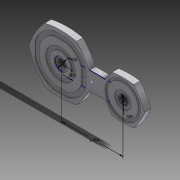
# Autodesk Inventor part: Frame
Saved by Autodesk Inventor 2018 (Build 220112000, 112)
## iProperties
Created: 2018-01-20
Part Number: Frame
Material: ABS Plastic
Document SubType Name: Modeling
Designer: Rus
Density: 1.06 g/cm^3
Appearance: Smooth - White
Author: Rus
Autodesk Inventor part; units mm, degrees
ref_plane "YZ Plane" through (0, 0, 0) normal (1, 0, 0) x (0, 1, 0)
ref_plane "XZ Plane" through (0, 0, 0) normal (0, 1, 0) x (-1, 0, 0)
ref_plane "XY Plane" through (0, 0, 0) normal (0, 0, 1) x (1, 0, 0)
sketch "Sketch1" plane through (0, 0, 0) normal (0, 0, 1) x (1, 0, 0)
  circle A0 centre (-43.9941, 0) radius 9.525
  circle A1 centre (43.9941, 0) radius 6.35
  line L0 (43.9941, 0) -> (-43.9941, 0) construction
  line L1 (43.9941, 12.7) -> (-43.9941, 12.7)
  line L2 (-43.9941, -12.7) -> (43.9941, -12.7)
  arc A2 (43.9941, -12.7) -> (43.9941, 12.7) centre (43.9941, 0) ccw
  arc A3 (-43.9941, 12.7) -> (-43.9941, -12.7) centre (-43.9941, 0) ccw
  point P0 (0, 0)
  point P1 (0, 0)
  dimension "d10" = 12.7
  dimension "d11" = 19.05
  dimension "d12" = 87.9881
  dimension "d13" = 12.7
  constraints: 8 end point, 4 centre point, 4 point on circle, 4 tangent, 1 coincident, 1 horizontal, 1 midpoint, 1 parallel
  measures "d10" diameter of A1
  measures "d11" diameter of A0
  measures "d12" distance of L0.start L0.end
  measures "d13" distance of L2.start L0.end
sketch "Sketch3" plane through (0, 0, 0) normal (0, 0, 1) x (1, 0, 0)
  line L0 (-44.9008, 0) -> (44.9008, 0) construction
  line L1 (-44.9008, -12.7) -> (44.9008, -12.7)
  line L2 (44.9008, 12.7) -> (-44.9008, 12.7)
  arc A0 (-44.9008, 12.7) -> (-44.9008, -12.7) centre (-44.9008, 0) ccw
  arc A1 (44.9008, -12.7) -> (44.9008, 12.7) centre (44.9008, 0) ccw
  circle A2 centre (-44.9008, 0) radius 6.35
  point P0 (0, 0)
  dimension "d23" = 44.9008
  dimension "d24" = 25.4
  dimension "d25" = 12.7
  constraints: 8 end point, 4 point on circle, 4 tangent, 3 centre point, 1 coincident, 1 horizontal, 1 midpoint, 1 parallel
  measures "d23" distance of point (0, 0) L0.end
  measures "d24" distance between parallel lines of L1 L2
  measures "d25" diameter of A2
extrude "Extrusion4" add sketch "Sketch3" against normal blind 8.4667
sketch "Sketch4" plane through (0, 0, -8.4667) normal (0, 0, -1) x (-1, 0, 0)
  circle A0 centre (-44.9008, 0) radius 6.35
  arc A1 (-44.9008, 12.7) -> (-44.9008, -12.7) centre (-44.9008, 0) ccw projected
  point P0 (0, 0)
  dimension "d28" = 12.7
  constraints: 1 centre point, 1 coincident
  measures "d28" diameter of A0
extrude "Extrusion5" cut sketch "Sketch4" against normal through all
sketch "Sketch5" plane through (0, 0, -8.4667) normal (0, 0, -1) x (-1, 0, 0)
  circle A0 centre (44.9008, 0) radius 6.35 projected
  line L0 (67.7609, 39.5947) -> (90.6209, 0)
  line L1 (90.6209, 0) -> (67.7608, -39.5947)
  line L2 (67.7608, -39.5947) -> (22.0408, -39.5947)
  line L3 (22.0408, -39.5947) -> (-0.8192, 0)
  line L4 (-0.8192, 0) -> (22.0409, 39.5947)
  line L5 (22.0409, 39.5947) -> (67.7609, 39.5947)
  line L6 (-44.9008, 12.7) -> (44.9008, 12.7) projected
  point P0 (0, 0)
  dimension "d31" = 45.72
  constraints: 12 end point, 2 coincident, 1 parallel, 13 other
  measures "d31" distance of L4.end L0.start
extrude "Extrusion6" add sketch "Sketch5" against normal up to surface (8.4667 mm away)
sketch "Sketch6" plane through (0, 0, 0) normal (0, 0, 1) x (1, 0, 0)
  line L0 (-52.1227, 63.088) -> (-51.6134, 26.2115) projected
  arc A0 (-51.6134, 26.2115) -> (-38.9146, 26.3869) centre (-45.264, 26.2992) ccw projected
  line L1 (-38.9146, 26.3869) -> (-39.4239, 63.2634) projected
  arc A1 (-26.5904, 60.8028) -> (-39.4239, 63.2634) centre (-44.9009, 0) ccw projected
  arc A2 (-26.5904, 60.8028) -> (15.3735, 19.9814) centre (17.7163, 64.3696) ccw projected
  arc A3 (18.1873, 7.2206) -> (15.3735, 19.9814) centre (-44.9009, 0) ccw projected
  line L2 (18.1873, 7.2206) -> (-18.6893, 6.7126) projected
  arc A4 (-18.6893, 6.7126) -> (-18.514, -5.9862) centre (-18.6017, 0.3632) ccw projected
  line L3 (-18.514, -5.9862) -> (18.3625, -5.4769) projected
  arc A5 (15.9019, -18.3105) -> (18.3625, -5.4769) centre (-44.9009, 0) ccw projected
  arc A6 (15.9019, -18.3105) -> (-24.9195, -60.2743) centre (19.4687, -62.6171) ccw projected
  arc A7 (-37.679, -63.088) -> (-24.9195, -60.2743) centre (-44.9009, 0) ccw projected
  line L4 (-37.679, -63.088) -> (-38.1883, -26.2115) projected
  arc A8 (-38.1883, -26.2115) -> (-50.8871, -26.3869) centre (-44.5377, -26.2992) ccw projected
  line L5 (-50.8871, -26.3869) -> (-50.3778, -63.2634) projected
  arc A9 (-63.2113, -60.8028) -> (-50.3778, -63.2634) centre (-44.9009, 0) ccw projected
  arc A10 (-63.2113, -60.8028) -> (-105.1752, -19.9814) centre (-107.518, -64.3696) ccw projected
  arc A11 (-107.9888, -7.2218) -> (-105.1752, -19.9814) centre (-44.9009, 0) ccw projected
  line L6 (-107.9888, -7.2218) -> (-71.1124, -6.7126) construction
  arc A12 (-71.1124, -6.7126) -> (-71.2877, 5.9862) centre (-71.2, -0.3632) ccw projected
  line L7 (-71.2877, 5.9862) -> (-108.1642, 5.4769) projected
  arc A13 (-105.7036, 18.3105) -> (-108.1642, 5.4769) centre (-44.9009, 0) ccw projected
  arc A14 (-105.7036, 18.3105) -> (-64.8822, 60.2743) centre (-109.2704, 62.6171) ccw projected
  arc A15 (-52.1227, 63.088) -> (-64.8822, 60.2743) centre (-44.9009, 0) ccw projected
  arc A16 (-55.6968, 34.5475) -> (-79.7331, 9.8384) centre (-44.9009, 0) ccw projected
  arc A17 (-79.7331, 9.8384) -> (-78.5109, 9.4932) centre (-79.122, 9.6658) ccw projected
  arc A18 (-55.318, 33.3353) -> (-78.5109, 9.4932) centre (-44.9009, 0) ccw projected
  arc A19 (-55.318, 33.3353) -> (-55.6968, 34.5475) centre (-55.5074, 33.9414) ccw projected
  arc A20 (-79.4483, -10.7959) -> (-54.7393, -34.8322) centre (-44.9009, 0) ccw projected
  arc A21 (-54.7393, -34.8322) -> (-54.3941, -33.61) centre (-54.5667, -34.2211) ccw projected
  arc A22 (-78.2361, -10.4171) -> (-54.3941, -33.61) centre (-44.9009, 0) ccw projected
  arc A23 (-78.2361, -10.4171) -> (-79.4483, -10.7959) centre (-78.8422, -10.6065) ccw projected
  arc A24 (-34.1049, -34.5475) -> (-10.0686, -9.8384) centre (-44.9009, 0) ccw projected
  arc A25 (-10.0686, -9.8384) -> (-11.2908, -9.4932) centre (-10.6797, -9.6658) ccw projected
  arc A26 (-34.4837, -33.3353) -> (-11.2908, -9.4932) centre (-44.9009, 0) ccw projected
  arc A27 (-34.4837, -33.3353) -> (-34.1049, -34.5475) centre (-34.2943, -33.9414) ccw projected
  arc A28 (-10.3534, 10.7959) -> (-35.0624, 34.8322) centre (-44.9009, 0) ccw projected
  arc A29 (-35.0624, 34.8322) -> (-35.4076, 33.61) centre (-35.235, 34.2211) ccw projected
  arc A30 (-11.5656, 10.4171) -> (-35.4076, 33.61) centre (-44.9009, 0) ccw projected
  arc A31 (-11.5656, 10.4171) -> (-10.3534, 10.7959) centre (-10.9595, 10.6065) ccw projected
  circle A32 centre (-44.9009, 0) radius 19.05 projected
  line L8 (-22.0408, -39.5947) -> (-67.7608, -39.5947) projected
  line L9 (-67.7609, -39.5947) -> (-90.6209, 0)
  line L10 (-90.6209, 0) -> (-67.7609, 39.5947)
  line L11 (-67.7609, 39.5947) -> (-22.0409, 39.5947)
  line L12 (-22.0409, 39.5947) -> (0.8191, 0)
  line L13 (0.8191, 0) -> (-22.0409, -39.5947)
  line L14 (-22.0409, -39.5947) -> (-67.7609, -39.5947)
  circle A33 centre (-44.9009, 0) radius 15.875
  circle A34 centre (-44.9009, 0) radius 17.78 projected
  circle A35 centre (-44.9009, 0) radius 9.525
  arc A36 (-54.7619, 36.8018) -> (-81.7026, 9.861) centre (-44.9009, 0) ccw
  line L15 (-44.9009, 0) -> (-71.8416, 26.9408) construction
  line L16 (-44.9009, 0) -> (-17.9601, 26.9408) construction
  arc A37 (-8.0991, 9.861) -> (-35.0398, 36.8018) centre (-44.9009, 0) ccw
  line L17 (-44.9009, 0) -> (-35.0398, 36.8018) construction
  line L18 (-44.9009, 0) -> (-6.8009, 0) construction
  line L19 (-54.7619, 36.8018) -> (-35.0398, 36.8018)
  line L20 (-67.7608, -39.5947) -> (-90.6209, 0) construction
  line L21 (-44.9009, 36.8018) -> (-90.6209, 0) construction
  line L22 (-81.7026, 9.861) -> (-81.5664, 0)
  line L23 (-44.9009, 0) -> (-81.5664, 0) construction
  line L24 (-8.0991, 9.861) -> (-8.0991, 0)
  arc A38 (-81.7026, -9.861) -> (-54.7619, -36.8018) centre (-44.9009, 0) ccw
  arc A39 (-35.0398, -36.8018) -> (-8.0991, -9.861) centre (-44.9009, 0) ccw
  line L25 (-54.7619, -36.8018) -> (-35.0398, -36.8018)
  line L26 (-81.7026, -9.861) -> (-81.5664, 0)
  line L27 (-8.0991, -9.861) -> (-8.0991, 0)
  circle A40 centre (-44.9009, 0) radius 21.1667
  arc A41 (-75.9187, -6.779) -> (-75.1884, -9.525) centre (-44.9009, 0) ccw construction
  line L28 (-75.1884, -9.525) -> (-75.1884, 9.525)
  line L29 (-54.4259, 30.2876) -> (-35.3758, 30.2876)
  line L30 (-14.6133, 9.525) -> (-14.6133, -9.525)
  line L31 (-35.3759, -30.2876) -> (-54.4259, -30.2876)
  arc A42 (-81.7026, 9.861) -> (-81.7026, -9.861) centre (-44.9009, 0) ccw construction
  line L32 (-76.6509, 0) -> (-75.1884, 0) construction
  arc A43 (-76.6509, 0) -> (-75.9187, -6.779) centre (-44.9009, 0) ccw construction
  arc A44 (-75.1884, -9.525) -> (-75.1884, 9.525) centre (-44.9009, 0) ccw
  arc A45 (-76.0941, 5.9198) -> (-76.6509, 0) centre (-44.9009, 0) ccw construction
  arc A46 (-75.1884, 9.525) -> (-76.0941, 5.9198) centre (-44.9009, 0) ccw
  point P0 (0, 0)
  point P1 (-44.9008, -39.5947)
  dimension "d43" = 63.5
  dimension "d34" = 31.75
  dimension "d35" = 19.05
  dimension "d36" = 60
  dimension "d37" = 38.1
  dimension "d38" = 38.1
  dimension "d40" = 60
  dimension "d41" = 90
  dimension "d42" = 42.3333
  dimension "d44" = 19.05
  dimension "d45" = 19.05
  constraints: 46 end point, 30 point on circle, 11 centre point, 9 coincident, 5 point on line, 4 horizontal, 4 midpoint, 4 symmetric about line, 3 equal length, 3 perpendicular, 2 parallel, 37 other
  measures "d34" diameter of A33
  measures "d35" diameter of A35
  measures "d37" radius of A36
  measures "d38" radius of A37
  measures "d41" angle of L16 L15
  measures "d42" diameter of A40
  measures "d44" distance of L31.start L31.end
  measures "d45" distance of L28.start L28.end
extrude "Extrusion7" add sketch "Sketch6" along normal blind 0.8467 contours L11 L1 L19 L0 | L0 L19 A36 L22 L7 L10 L11 | L11 L12 L2 L24 A37 L19 L1 | L7 L22 L26 A38 L25 L5 L8 L9 L10 | L29 L1 A0 A40 L0 | L0 A0 A40 A12 L7 L28 A44 L29 | L12 L13 L3 L27 L24 L2 | L29 A44 L30 L2 A4 A40 A0 L1 | L7 A12 A40 A8 L5 L31 A44 L28 | L5 L25 L4 L8 | L13 L8 L4 L25 A39 L27 L3 | L30 L3 A4 A40 L2 | L30 A44 L31 L4 A8 A40 A4 L3 | A40 A8 L4 L31 L5 | A33
sketch "Sketch7" plane through (0, 0, -8.4667) normal (0, 0, -1) x (-1, 0, 0)
  circle A0 centre (-44.9008, 0) radius 6.35 projected
  circle A1 centre (-44.9008, 0) radius 12.7
  line L0 (-44.9008, -12.7) -> (6.5132, -12.7) projected
  line L1 (-76.0633, 0) -> (-60.4821, 26.9875)
  line L2 (-60.4821, 26.9875) -> (-29.3196, 26.9875)
  line L3 (-29.3196, 26.9875) -> (-13.7384, 0)
  line L4 (-13.7384, 0) -> (-29.3196, -26.9875)
  line L5 (-29.3196, -26.9875) -> (-60.4821, -26.9875)
  line L6 (-60.4821, -26.9875) -> (-76.0633, 0)
  arc A2 (-60.4821, 26.9875) -> (-76.0633, 0) centre (18.6746, -36.7053) ccw
  arc A3 (-76.0633, 0) -> (-60.4821, -26.9875) centre (18.6746, 36.7053) ccw
  arc A4 (-60.4821, -26.9875) -> (-29.3196, -26.9875) centre (-44.9009, 73.4106) ccw
  arc A5 (-29.3196, -26.9875) -> (-13.7384, 0) centre (-108.4763, 36.7053) ccw
  arc A6 (-13.7384, 0) -> (-29.3196, 26.9875) centre (-108.4763, -36.7053) ccw
  arc A7 (-29.3196, 26.9875) -> (-60.4821, 26.9875) centre (-44.9008, -73.4106) ccw
  point P0 (0, 0)
  point P1 (5.3062, -12.7)
  dimension "d48" = 53.975
  dimension "d49" = 101.6
  dimension "d50" = 101.6
  dimension "d51" = 101.6
  dimension "d52" = 101.6
  dimension "d53" = 101.6
  dimension "d54" = 101.6
  constraints: 13 end point, 12 point on circle, 7 centre point, 2 coincident, 1 horizontal, 1 tangent, 13 other
  measures "d48" distance between parallel lines of L5 L2
  measures "d49" radius of A2
  measures "d50" radius of A3
  measures "d51" radius of A4
  measures "d52" radius of A5
  measures "d53" radius of A6
  measures "d54" radius of A7
extrude "Extrusion8" add sketch "Sketch7" against normal up to surface (8.4667 mm away) contours L4 A5 L0 | L4 L5 L6 L1 L2 L3 | L0 A5 L4 | L3 A6 | A4 L5 | L2 A7 | A3 L6 | L1 A2
sketch "Sketch8" plane through (0, 0, -8.4667) normal (0, 0, -1) x (-1, 0, 0)
  line L0 (22.0409, 39.5947) -> (67.7609, 39.5947) construction
  line L1 (22.0409, 39.5947) -> (67.7609, 39.5947) construction
  arc A0 (67.7609, 39.5947) -> (22.0409, 39.5947) centre (44.9008, -59.4002) ccw
  line L2 (6.5132, 12.7) -> (22.0409, 39.5947) construction
  line L3 (22.0408, -39.5947) -> (6.5132, -12.7) construction
  line L4 (67.7608, -39.5947) -> (22.0408, -39.5947) construction
  arc A1 (22.0408, -39.5947) -> (67.7608, -39.5947) centre (44.9009, 59.4002) ccw
  line L5 (90.6209, 0) -> (67.7608, -39.5947) construction
  arc A2 (67.7608, -39.5947) -> (90.6209, 0) centre (-6.5412, 29.7001) ccw
  line L6 (67.7609, 39.5947) -> (90.6209, 0) construction
  arc A3 (90.6209, 0) -> (67.7609, 39.5947) centre (-6.5412, -29.7001) ccw
  arc A4 (22.0409, 39.5947) -> (-0.8192, 0) centre (96.3429, -29.7001) ccw
  line L7 (67.7608, -39.5947) -> (22.0408, -39.5947) construction
  arc A5 (-0.8192, 0) -> (22.0408, -39.5947) centre (96.3429, 29.7001) ccw
  circle A6 centre (44.9009, 0) radius 9.525 projected
  line L8 (90.6209, 0) -> (67.7609, -39.5947)
  line L9 (67.7609, -39.5947) -> (22.0409, -39.5947)
  line L10 (22.0409, -39.5947) -> (-0.8191, 0)
  line L11 (-0.8191, 0) -> (22.0409, 39.5947)
  line L12 (22.0409, 39.5947) -> (67.7608, 39.5947)
  line L13 (67.7608, 39.5947) -> (90.6209, 0)
  point P0 (0, 0)
  point P1 (5.3062, 12.7)
  point P2 (5.3062, -12.7)
  dimension "d57" = 101.6
  constraints: 12 end point, 12 point on circle, 6 centre point, 5 equal radius, 2 point on line, 1 coincident, 15 other
  measures "d57" radius of A3
extrude "Extrusion9" add sketch "Sketch8" against normal up to surface (9.3133 mm away) contours L12 A0 | A3 L13 | L11 A4 | A2 L8 | L10 A5 | A1 L9
sketch "Sketch9" plane through (0, 0, 0) normal (0, 0, 1) x (1, 0, 0)
  circle A0 centre (44.9008, 0) radius 6.35 projected
  line L0 (19.6975, 12.7) -> (-4.0131, 12.7) projected
  line L1 (-4.0131, -12.7) -> (19.6975, -12.7) projected
  arc A1 (19.6975, -12.7) -> (29.3196, -26.9875) centre (108.4763, 36.7053) ccw projected
  arc A2 (29.3196, -26.9875) -> (60.4821, -26.9875) centre (44.9009, 73.4106) ccw projected
  arc A3 (60.4821, -26.9875) -> (76.0633, 0) centre (-18.6746, 36.7053) ccw projected
  arc A4 (76.0633, 0) -> (60.4821, 26.9875) centre (-18.6746, -36.7053) ccw projected
  arc A5 (60.4821, 26.9875) -> (29.3196, 26.9875) centre (44.9008, -73.4106) ccw projected
  arc A6 (29.3196, 26.9875) -> (19.6975, 12.7) centre (108.4763, -36.7053) ccw projected
  circle A7 centre (44.9008, 0) radius 25.4
  circle A8 centre (44.9008, 0) radius 22.0133
  circle A9 centre (44.9008, 0) radius 7.1967
  circle A10 centre (44.9008, 0) radius 11.8533
  arc A11 (-4.0131, -12.7) -> (0.8191, 0) centre (-96.3429, 29.7001) ccw projected
  arc A12 (0.8191, 0) -> (-4.0131, 12.7) centre (-96.3429, -29.7001) ccw projected
  point P0 (0, 0)
  dimension "d60" = 50.8
  dimension "d61" = 3.3867
  dimension "d62" = 0.8467
  dimension "d63" = 4.6567
  constraints: 4 centre point, 4 coincident
  measures "d60" diameter of A7
  measures "d61" radial gap between concentric circles of A8 A7
  measures "d62" radial gap between concentric circles of A9 A0
  measures "d63" radial gap between concentric circles of A9 A10
extrude "Extrusion10" add sketch "Sketch9" along normal up to surface (0.8467 mm away)
sketch "Sketch10" plane through (0, 0, 0.8467) normal (0, 0, 1) x (1, 0, 0)
  point P0 (0, 0)
body "Solid2"
